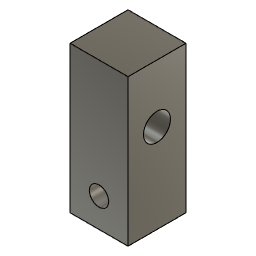
wall-E_standoff v1 (Autodesk Fusion 360 design; units mm, degrees)
Autodesk Fusion 360 part; units mm, degrees
note: some values were not read from the file. Set by a fixed rule: which sketch regions a step uses.
sketch "Sketch1" plane through (0, 0, 0) normal (0, 0, 1) x (1, 0, 0)
  line L0 (0, 0) -> (15, 0)
  line L1 (15, 0) -> (15, 15)
  line L2 (15, 15) -> (0, 15)
  line L3 (0, 15) -> (0, 0)
  dimension "d1" = 15
  dimension "d2" = 15
  constraint horizontal L0
  constraint vertical L1
  constraint horizontal L2
  constraint vertical L3
  constraint coincident L0.start L3.end
  measures "d1" distance of L0.start L0.end
  measures "d2" distance of L0.start L2.end
extrude "Extrude1" add sketch "Sketch1" along normal blind 35
extrude "Extrude2" add 1 faces at (5, 10, 35) along direction (0, 0, 1) blind 3
sketch "Sketch2" plane through (15, 0, 0) normal (1, 0, 0) x (0, 1, 0)
  line L0 (0, 0) -> (15, 0)
  line L1 (15, 0) -> (15, 38)
  line L2 (15, 38) -> (0, 38)
  line L3 (0, 38) -> (0, 0)
  line L4 (0, 38) -> (15, 38)
  line L5 (15, 38) -> (15, 35.5)
  line L6 (15, 35.5) -> (0, 35.5)
  line L7 (0, 35.5) -> (0, 38)
  line L8 (0, 35.5) -> (15, 35.5)
  line L9 (15, 35.5) -> (15, 30.5)
  line L10 (15, 30.5) -> (0, 30.5)
  line L11 (0, 30.5) -> (0, 35.5)
  line L12 (0, 30.5) -> (15, 30.5)
  line L13 (15, 30.5) -> (15, 15.5)
  line L14 (15, 15.5) -> (0, 15.5)
  line L15 (0, 15.5) -> (0, 30.5)
  line L16 (0, 30.5) -> (15, 15.5)
  line L17 (15, 30.5) -> (0, 15.5)
  circle A0 centre (7.5, 23) radius 3.5
  dimension "d7" = 2.5
  dimension "d8" = 5
  dimension "d9" = 15
  dimension "d10" = 7
  constraint horizontal L4
  constraint vertical L5
  constraint horizontal L6
  constraint vertical L7
  constraint coincident L1 L5.end
  constraint coincident L2.end L3.start
  constraint horizontal L8
  constraint vertical L9
  constraint horizontal L10
  constraint vertical L11
  constraint horizontal L12
  constraint vertical L13
  constraint horizontal L14
  constraint vertical L15
  constraint perpendicular L16 L17
  constraint midpoint L17 A0.centre
  measures "d7" distance of L1.end L5.end
  measures "d8" distance of L6.end L10.end
  measures "d9" distance of L10.end L14.end
  measures "d10" diameter of A0
extrude "Extrude3" cut sketch "Sketch2" against normal blind 45 contours L16 L17 A0 | L16 L17 A0 | L16 L17 A0 | L16 L17 A0
sketch "Sketch3" plane through (0, 0, 0) normal (0, -1, 0) x (1, 0, 0)
  line L0 (0, 0) -> (15, 0)
  line L1 (15, 0) -> (15, 38)
  line L2 (15, 38) -> (0, 38)
  line L3 (0, 38) -> (0, 0)
  line L4 (0, 0) -> (15, 0)
  line L5 (15, 0) -> (15, 15)
  line L6 (15, 15) -> (0, 15)
  line L7 (0, 15) -> (0, 0)
  line L8 (0, 15) -> (15, 0)
  line L9 (15, 15) -> (0, 0)
  circle A0 centre (7.5, 7.5) radius 2.5
  dimension "d13" = 15
  dimension "d14" = 15
  dimension "d15" = 5
  constraint horizontal L4
  constraint vertical L5
  constraint horizontal L6
  constraint vertical L7
  constraint coincident L0.start L3.end
  constraint coincident L0.end L1.start
  constraint midpoint L8 A0.centre
  measures "d13" distance of L0.start L0.end
  measures "d14" distance of L0.start L6.end
  measures "d15" diameter of A0
extrude "Extrude4" cut sketch "Sketch3" against normal blind 45 contours L8 L9 A0 | L8 L9 A0 | L8 L9 A0 | L8 L9 A0
